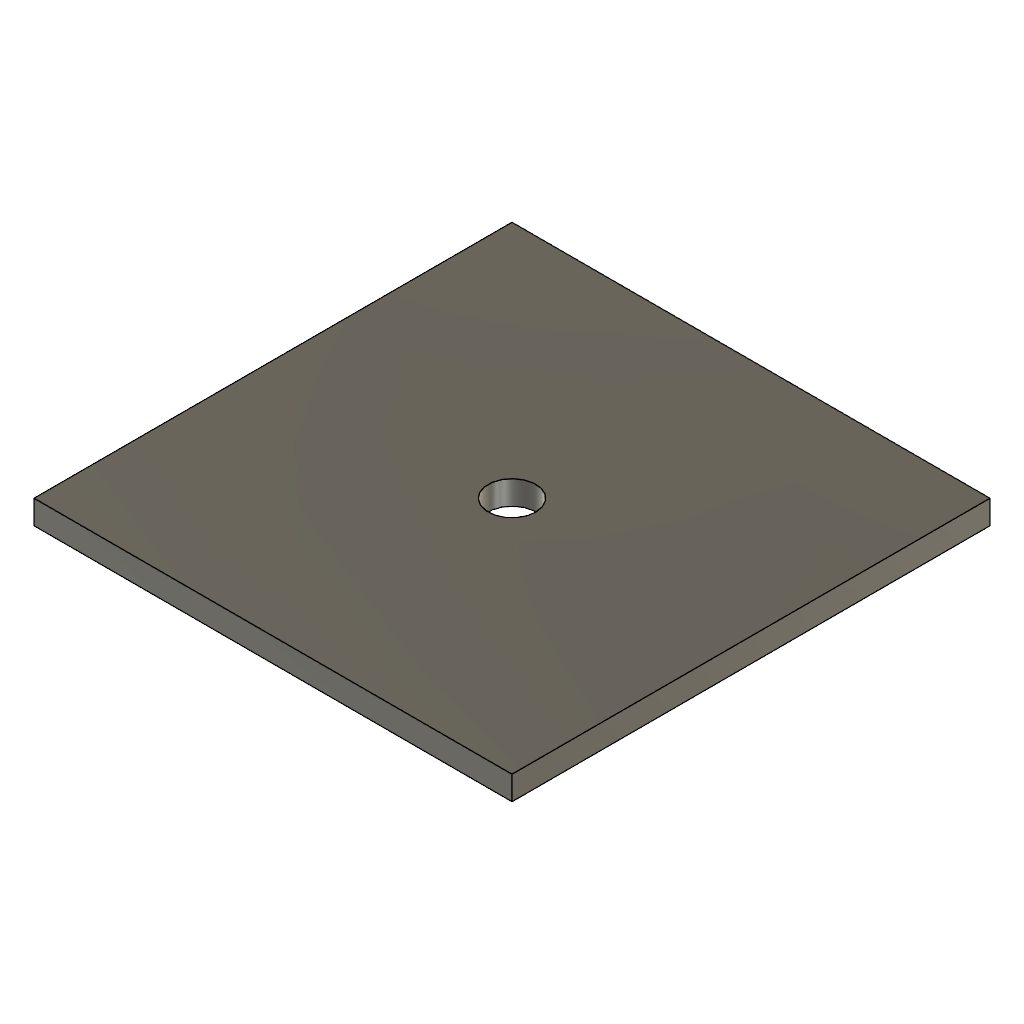
smart dice (Assembly) (Autodesk Fusion 360 archive; units mm, degrees)
design "steen ontwerp smart dice bovenkant"
Autodesk Fusion 360 part; units mm, degrees
sketch "Sketch1" plane through (0, 0, 0) normal (0, 0, 1) x (1, 0, 0)
  line L0 (-50, 50) -> (50, 50)
  line L1 (50, 50) -> (50, -50)
  line L2 (50, -50) -> (-50, -50)
  line L3 (-50, -50) -> (-50, 50)
  line L4 (-50, 50) -> (50, -50) construction
  line L5 (50, 50) -> (-50, -50) construction
  dimension "d1" = 100
  dimension "d2" = 100
  constraint horizontal L0
  constraint perpendicular L0 L1
  constraint parallel L0 L2
  constraint parallel L1 L3
  constraint coincident L4 origin
  constraint coincident L5 origin
  measures "d1" distance of L1.end L2.end
  measures "d2" distance of L0.end L1.end
extrude "Extrude1" add sketch "Sketch1" along normal blind 5
sketch "Sketch2" plane through (0, 0, 5) normal (0, 0, 1) x (-1, 0, 0)
  line L0 (50, 50) -> (-50, 50)
  line L1 (-50, 50) -> (-50, -50)
  line L2 (-50, -50) -> (50, -50)
  line L3 (50, -50) -> (50, 50)
  line L4 (40, -50) -> (40, 50) construction
  line L5 (30, -50) -> (30, 50) construction
  line L6 (20, 50) -> (20, -50) construction
  line L7 (10, -50) -> (10, 50) construction
  line L8 (0, 50) -> (0, -50) construction
  line L9 (-10, -50) -> (-10, 50) construction
  line L10 (-20, 50) -> (-20, -50) construction
  line L11 (-30, -50) -> (-30, 50) construction
  line L12 (-40, -50) -> (-40, 50) construction
  line L13 (-50, 40) -> (50, 40) construction
  line L14 (50, 30) -> (-50, 30) construction
  line L15 (-50, 20) -> (50, 20) construction
  line L16 (50, 10) -> (-50, 10) construction
  line L17 (-50, 0) -> (50, 0) construction
  line L18 (50, -10) -> (-50, -10) construction
  line L19 (-50, -20) -> (50, -20) construction
  line L20 (50, -30) -> (-50, -30) construction
  line L21 (-50, -40) -> (50, -40) construction
  circle A0 centre (0, 0) radius 5
  dimension "d5" = 10
  constraint coincident L2 L4.start
  constraint coincident L0 L4.end
  constraint perpendicular L0 L4
  constraint coincident L2 L5.start
  constraint coincident L0 L5.end
  constraint perpendicular L0 L5
  constraint coincident L0 L6.start
  constraint coincident L2 L6.end
  constraint perpendicular L2 L6
  constraint coincident L2 L7.start
  constraint coincident L0 L7.end
  constraint perpendicular L0 L7
  constraint midpoint L0 L8.start
  constraint midpoint L2 L8.end
  constraint coincident L2 L9.start
  constraint coincident L0 L9.end
  constraint perpendicular L0 L9
  constraint coincident L0 L10.start
  constraint coincident L2 L10.end
  constraint perpendicular L2 L10
  constraint coincident L2 L11.start
  constraint coincident L0 L11.end
  constraint perpendicular L0 L11
  constraint coincident L2 L12.start
  constraint coincident L0 L12.end
  constraint perpendicular L0 L12
  constraint coincident L1 L13.start
  constraint coincident L3 L13.end
  constraint perpendicular L3 L13
  constraint coincident L3 L14.start
  constraint coincident L1 L14.end
  constraint perpendicular L1 L14
  constraint coincident L1 L15.start
  constraint coincident L3 L15.end
  constraint perpendicular L3 L15
  constraint coincident L3 L16.start
  constraint coincident L1 L16.end
  constraint perpendicular L1 L16
  constraint midpoint L1 L17.start
  constraint midpoint L3 L17.end
  constraint coincident L3 L18.start
  constraint coincident L1 L18.end
  constraint perpendicular L1 L18
  constraint coincident L1 L19.start
  constraint coincident L3 L19.end
  constraint perpendicular L3 L19
  constraint coincident L3 L20.start
  constraint coincident L1 L20.end
  constraint perpendicular L1 L20
  constraint coincident L1 L21.start
  constraint coincident L3 L21.end
  constraint perpendicular L3 L21
  constraint coincident A0.centre origin
  measures "d5" diameter of A0
extrude "Extrude2" cut sketch "Sketch2" against normal blind 5 contours A0
sketch "Sketch3" plane through (0, 0, 0) normal (0, 0, -1) x (1, 0, 0)
  circle A0 centre (0, 0) radius 5
  line L0 (50, 50) -> (-50, 50)
  line L1 (-50, 50) -> (-50, -50)
  line L2 (-50, -50) -> (50, -50)
  line L3 (50, -50) -> (50, 50)
  line L4 (-50, 50) -> (-30, 50)
  line L5 (-30, -50) -> (-50, -50)
  line L6 (-50, -50) -> (-50, 50)
  line L7 (27.6819, -50) -> (50, -50)
  line L8 (50, -50) -> (50, 50)
  line L9 (50, 50) -> (27.6819, 50)
  line L10 (-40, 40) -> (-20, 40)
  line L11 (-20, 40) -> (-20, -40)
  line L12 (-20, -40) -> (-40, -40)
  line L13 (-40, -40) -> (-40, 40)
  line L14 (20, -40) -> (40, -40)
  line L15 (40, -40) -> (40, 40)
  line L16 (40, 40) -> (20, 40)
  line L17 (20, 40) -> (20, -40)
  constraint horizontal L4
  constraint horizontal L5
  constraint vertical L6
  constraint coincident L2 L5.start
  constraint coincident L0.end L1.start
  constraint horizontal L7
  constraint vertical L8
  constraint horizontal L9
  constraint coincident L0.start L3.end
  constraint coincident L2 L7.start
  constraint horizontal L10
  constraint vertical L11
  constraint horizontal L12
  constraint vertical L13
  constraint horizontal L14
  constraint vertical L15
  constraint horizontal L16
  constraint vertical L17
extrude "Extrude3" cut sketch "Sketch3" against normal blind 2 contours L10 L11 L12 L13 | L14 L15 L16 L17

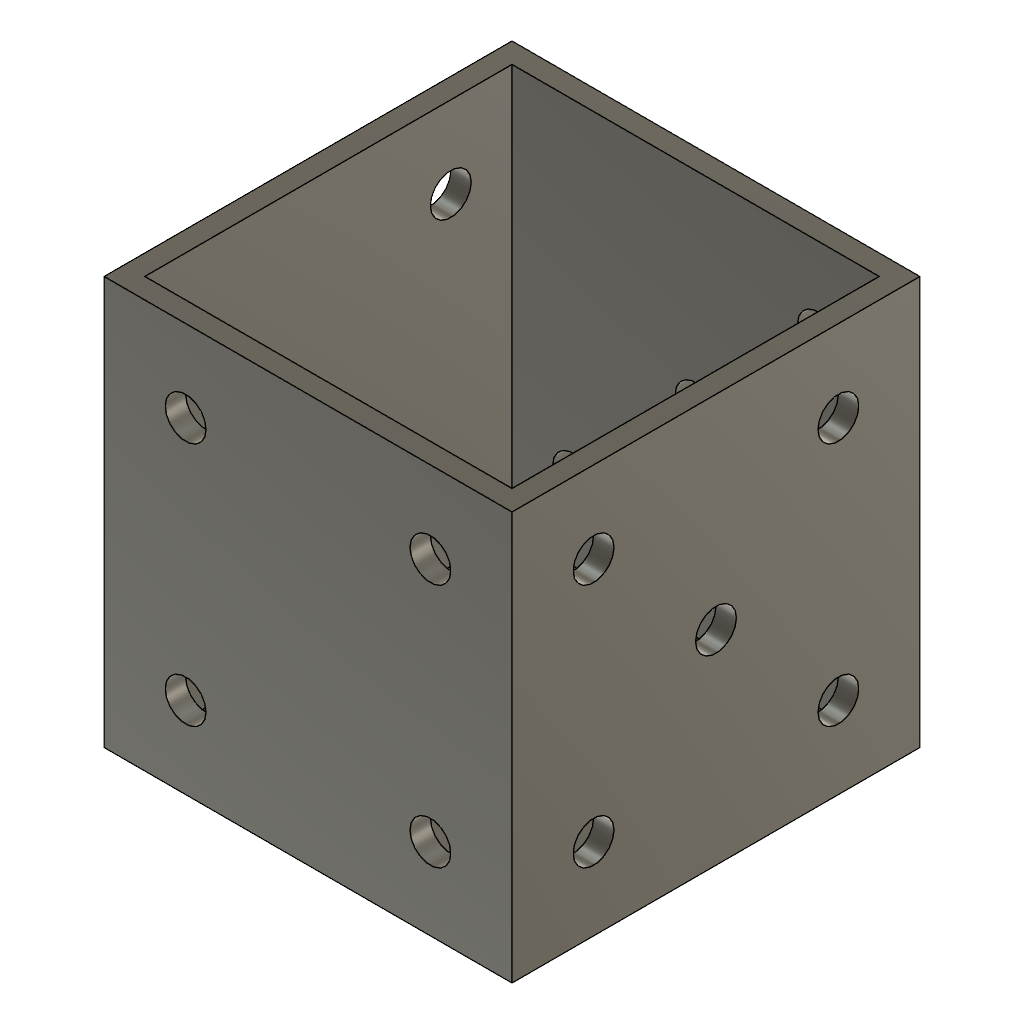
design "steen ontwerp smart dice onderkant"
Autodesk Fusion 360 part; units mm, degrees
sketch "Sketch1" plane through (0, 0, 0) normal (0, 0, 1) x (1, 0, 0)
  line L0 (-50, 50) -> (50, 50)
  line L1 (50, 50) -> (50, -50)
  line L2 (50, -50) -> (-50, -50)
  line L3 (-50, -50) -> (-50, 50)
  line L4 (-45, -45) -> (45, -45)
  line L5 (45, -45) -> (45, 45)
  line L6 (45, 45) -> (-45, 45)
  line L7 (-45, 45) -> (-45, -45)
  line L8 (-45, -45) -> (45, 45) construction
  line L9 (45, -45) -> (-45, 45) construction
  dimension "d5" = 90
  dimension "d6" = 90
  constraint horizontal L0
  constraint vertical L1
  constraint horizontal L2
  constraint vertical L3
  constraint horizontal L4
  constraint perpendicular L4 L5
  constraint parallel L4 L6
  constraint parallel L5 L7
  constraint coincident L8 origin
  constraint coincident L9 origin
  measures "d5" distance of L5.end L6.end
  measures "d6" distance of L4.end L5.end
extrude "Extrude3" add sketch "Sketch1" along normal blind 100
extrude "Extrude4" add sketch "Sketch1" along normal blind 1 contours L4 L5 L6 L7
sketch "Sketch3" plane through (50, 0, 0) normal (1, 0, 0) x (0, 1, 0)
  line L0 (-50, 0) -> (50, 0)
  line L1 (50, 0) -> (50, 100)
  line L2 (50, 100) -> (-50, 100)
  line L3 (-50, 100) -> (-50, 0)
  line L4 (-40, 100) -> (-40, 0) construction
  line L5 (-30, 100) -> (-30, 0) construction
  line L6 (-20, 100) -> (-20, 0) construction
  line L7 (-10, 100) -> (-10, 0) construction
  line L8 (10, 100) -> (10, 0) construction
  line L9 (20, 100) -> (20, 0) construction
  line L10 (30, 100) -> (30, 0) construction
  line L11 (40, 100) -> (40, 0) construction
  line L12 (-50, 10) -> (50, 10) construction
  line L13 (-50, 20) -> (50, 20) construction
  line L14 (-50, 30) -> (50, 30) construction
  line L15 (-50, 40) -> (50, 40) construction
  line L16 (-50, 50) -> (50, 50) construction
  line L17 (-50, 60) -> (50, 60) construction
  line L18 (-50, 70) -> (50, 70) construction
  line L19 (50, 80) -> (-50, 80) construction
  line L20 (-50, 90) -> (50, 90) construction
  line L21 (0, 100) -> (0, 0) construction
  circle A0 centre (-30, 80) radius 5
  circle A1 centre (30, 80) radius 5
  circle A2 centre (-30, 20) radius 5
  circle A3 centre (30, 20) radius 5
  circle A4 centre (0, 50) radius 5
  dimension "d12" = 10
  dimension "d13" = 10
  dimension "d14" = 10
  dimension "d15" = 10
  dimension "d16" = 10
  constraint coincident L2 L4.start
  constraint coincident L0 L4.end
  constraint perpendicular L0 L4
  constraint coincident L2 L5.start
  constraint coincident L0 L5.end
  constraint perpendicular L0 L5
  constraint coincident L2 L6.start
  constraint coincident L0 L6.end
  constraint perpendicular L0 L6
  constraint coincident L2 L7.start
  constraint coincident L0 L7.end
  constraint perpendicular L0 L7
  constraint coincident L2 L8.start
  constraint coincident L0 L8.end
  constraint perpendicular L0 L8
  constraint coincident L2 L9.start
  constraint coincident L0 L9.end
  constraint perpendicular L0 L9
  constraint coincident L2 L10.start
  constraint coincident L0 L10.end
  constraint perpendicular L0 L10
  constraint coincident L2 L11.start
  constraint coincident L0 L11.end
  constraint perpendicular L0 L11
  constraint coincident L3 L12.start
  constraint coincident L1 L12.end
  constraint perpendicular L1 L12
  constraint coincident L3 L13.start
  constraint coincident L1 L13.end
  constraint perpendicular L1 L13
  constraint coincident L3 L14.start
  constraint coincident L1 L14.end
  constraint perpendicular L1 L14
  constraint coincident L3 L15.start
  constraint coincident L1 L15.end
  constraint perpendicular L1 L15
  constraint midpoint L3 L16.start
  constraint midpoint L1 L16.end
  constraint coincident L3 L17.start
  constraint coincident L1 L17.end
  constraint perpendicular L1 L17
  constraint coincident L3 L18.start
  constraint coincident L1 L18.end
  constraint perpendicular L1 L18
  constraint coincident L1 L19.start
  constraint coincident L3 L19.end
  constraint perpendicular L3 L19
  constraint coincident L3 L20.start
  constraint coincident L1 L20.end
  constraint perpendicular L1 L20
  constraint midpoint L2 L21.start
  constraint coincident L21.end origin
  constraint coincident L19 A0.centre
  constraint coincident L5 A0.centre
  constraint coincident L10 A1.centre
  constraint coincident L19 A1.centre
  constraint coincident L5 A2.centre
  constraint coincident L13 A2.centre
  constraint coincident L10 A3.centre
  constraint coincident L13 A3.centre
  constraint midpoint L21 A4.centre
  measures "d12" diameter of A0
  measures "d13" diameter of A1
  measures "d14" diameter of A2
  measures "d15" diameter of A3
  measures "d16" diameter of A4
extrude "Extrude5" cut sketch "Sketch3" against normal blind 10 contours A0 | A1 | A2 | A3 | A4
sketch "Sketch4" plane through (-50, 0, 0) normal (-1, 0, 0) x (0, -1, 0)
  line L0 (-50, 0) -> (50, 0)
  line L1 (50, 0) -> (50, 100)
  line L2 (50, 100) -> (-50, 100)
  line L3 (-50, 100) -> (-50, 0)
  line L4 (-40, 100) -> (-40, 0) construction
  line L5 (-30, 0) -> (-30, 100) construction
  line L6 (-20, 100) -> (-20, 0) construction
  line L7 (-10, 0) -> (-10, 100) construction
  line L8 (0, 100) -> (0, 0) construction
  line L9 (10, 0) -> (10, 100) construction
  line L10 (20, 100) -> (20, 0) construction
  line L11 (30, 0) -> (30, 100) construction
  line L12 (40, 100) -> (40, 0) construction
  line L13 (50, 10) -> (-50, 10) construction
  line L14 (-50, 20) -> (50, 20) construction
  line L15 (50, 30) -> (-50, 30) construction
  line L16 (-50, 40) -> (50, 40) construction
  line L17 (50, 50) -> (-50, 50) construction
  line L18 (-50, 60) -> (50, 60) construction
  line L19 (50, 70) -> (-50, 70) construction
  line L20 (-50, 80) -> (50, 80) construction
  line L21 (50, 90) -> (-50, 90) construction
  circle A0 centre (-30, 80) radius 5
  circle A1 centre (30, 20) radius 5
  dimension "d19" = 10
  dimension "d20" = 10
  constraint coincident L2 L4.start
  constraint coincident L0 L4.end
  constraint perpendicular L0 L4
  constraint coincident L0 L5.start
  constraint coincident L2 L5.end
  constraint perpendicular L2 L5
  constraint coincident L2 L6.start
  constraint coincident L0 L6.end
  constraint perpendicular L0 L6
  constraint coincident L0 L7.start
  constraint coincident L2 L7.end
  constraint perpendicular L2 L7
  constraint midpoint L2 L8.start
  constraint coincident L8.end origin
  constraint coincident L0 L9.start
  constraint coincident L2 L9.end
  constraint perpendicular L2 L9
  constraint coincident L2 L10.start
  constraint coincident L0 L10.end
  constraint perpendicular L0 L10
  constraint coincident L0 L11.start
  constraint coincident L2 L11.end
  constraint perpendicular L2 L11
  constraint coincident L2 L12.start
  constraint coincident L0 L12.end
  constraint perpendicular L0 L12
  constraint coincident L1 L13.start
  constraint coincident L3 L13.end
  constraint perpendicular L3 L13
  constraint coincident L3 L14.start
  constraint coincident L1 L14.end
  constraint perpendicular L1 L14
  constraint coincident L1 L15.start
  constraint coincident L3 L15.end
  constraint perpendicular L3 L15
  constraint coincident L3 L16.start
  constraint coincident L1 L16.end
  constraint perpendicular L1 L16
  constraint midpoint L1 L17.start
  constraint midpoint L3 L17.end
  constraint coincident L3 L18.start
  constraint coincident L1 L18.end
  constraint perpendicular L1 L18
  constraint coincident L1 L19.start
  constraint coincident L3 L19.end
  constraint perpendicular L3 L19
  constraint coincident L3 L20.start
  constraint coincident L1 L20.end
  constraint perpendicular L1 L20
  constraint coincident L1 L21.start
  constraint coincident L3 L21.end
  constraint perpendicular L3 L21
  constraint coincident L20 A0.centre
  constraint coincident L5 A0.centre
  constraint coincident L11 A1.centre
  constraint coincident L14 A1.centre
  measures "d19" diameter of A0
  measures "d20" diameter of A1
extrude "Extrude6" cut sketch "Sketch4" against normal blind 10 contours A0
extrude "Extrude7" cut sketch "Sketch4" against normal blind 10 contours A1
sketch "Sketch5" plane through (0, 0, 0) normal (0, 0, -1) x (1, 0, 0)
  line L0 (50, 50) -> (-50, 50)
  line L1 (-50, 50) -> (-50, -50)
  line L2 (-50, -50) -> (50, -50)
  line L3 (50, -50) -> (50, 50)
  line L4 (-40, 50) -> (-40, -50) construction
  line L5 (-30, -50) -> (-30, 50) construction
  line L6 (-20, 50) -> (-20, -50) construction
  line L7 (-10, -50) -> (-10, 50) construction
  line L8 (0, 50) -> (0, -50) construction
  line L9 (10, -50) -> (10, 50) construction
  line L10 (20, 50) -> (20, -50) construction
  line L11 (30, -50) -> (30, 50) construction
  line L12 (40, 50) -> (40, -50) construction
  line L13 (50, -40) -> (-50, -40) construction
  line L14 (-50, -30) -> (50, -30) construction
  line L15 (50, -20) -> (-50, -20) construction
  line L16 (-50, -10) -> (50, -10) construction
  line L17 (50, 0) -> (-50, 0) construction
  line L18 (-50, 10) -> (50, 10) construction
  line L19 (50, 20) -> (-50, 20) construction
  line L20 (-50, 30) -> (50, 30) construction
  line L21 (-50, 40) -> (50, 40) construction
  circle A0 centre (-30, 30) radius 5
  circle A1 centre (30, 30) radius 5
  circle A2 centre (-30, 0) radius 5
  circle A3 centre (30, 0) radius 5
  circle A4 centre (-30, -30) radius 5
  circle A5 centre (30, -30) radius 5
  dimension "d25" = 10
  dimension "d26" = 10
  dimension "d27" = 10
  dimension "d28" = 10
  dimension "d29" = 10
  dimension "d30" = 10
  constraint coincident L0 L4.start
  constraint coincident L2 L4.end
  constraint perpendicular L2 L4
  constraint coincident L2 L5.start
  constraint coincident L0 L5.end
  constraint perpendicular L0 L5
  constraint coincident L0 L6.start
  constraint coincident L2 L6.end
  constraint perpendicular L2 L6
  constraint coincident L2 L7.start
  constraint coincident L0 L7.end
  constraint perpendicular L0 L7
  constraint midpoint L0 L8.start
  constraint midpoint L2 L8.end
  constraint coincident L2 L9.start
  constraint coincident L0 L9.end
  constraint perpendicular L0 L9
  constraint coincident L0 L10.start
  constraint coincident L2 L10.end
  constraint perpendicular L2 L10
  constraint coincident L2 L11.start
  constraint coincident L0 L11.end
  constraint perpendicular L0 L11
  constraint coincident L0 L12.start
  constraint coincident L2 L12.end
  constraint perpendicular L2 L12
  constraint coincident L3 L13.start
  constraint coincident L1 L13.end
  constraint perpendicular L1 L13
  constraint coincident L1 L14.start
  constraint coincident L3 L14.end
  constraint perpendicular L3 L14
  constraint coincident L3 L15.start
  constraint coincident L1 L15.end
  constraint perpendicular L1 L15
  constraint coincident L1 L16.start
  constraint coincident L3 L16.end
  constraint perpendicular L3 L16
  constraint midpoint L3 L17.start
  constraint midpoint L1 L17.end
  constraint coincident L1 L18.start
  constraint coincident L3 L18.end
  constraint perpendicular L3 L18
  constraint coincident L3 L19.start
  constraint coincident L1 L19.end
  constraint coincident L1 L20.start
  constraint coincident L3 L20.end
  constraint perpendicular L3 L20
  constraint coincident L1 L21.start
  constraint coincident L3 L21.end
  constraint perpendicular L3 L21
  constraint coincident L5 A0.centre
  constraint coincident L20 A0.centre
  constraint coincident L11 A1.centre
  constraint coincident L20 A1.centre
  constraint midpoint L5 A2.centre
  constraint midpoint L11 A3.centre
  constraint coincident L14 A4.centre
  constraint coincident L5 A4.centre
  constraint coincident L14 A5.centre
  constraint coincident L11 A5.centre
  measures "d25" diameter of A0
  measures "d26" diameter of A1
  measures "d27" diameter of A2
  measures "d28" diameter of A3
  measures "d29" diameter of A4
  measures "d30" diameter of A5
extrude "Extrude8" cut sketch "Sketch5" against normal blind 2 contours A0 | A1 | A2 | A3 | A4 | A5
sketch "Sketch7" plane through (0, -50, 0) normal (0, -1, 0) x (1, 0, 0)
  line L0 (-50, 0) -> (50, 0)
  line L1 (50, 0) -> (50, 100)
  line L2 (50, 100) -> (-50, 100)
  line L3 (-50, 100) -> (-50, 0)
  line L4 (-40, 100) -> (-40, 0) construction
  line L5 (-30, 0) -> (-30, 100) construction
  line L6 (-20, 100) -> (-20, 0) construction
  line L7 (-10, 0) -> (-10, 100) construction
  line L8 (0, 100) -> (0, 0) construction
  line L9 (10, 0) -> (10, 100) construction
  line L10 (20, 0) -> (20, 100) construction
  line L11 (30, 100) -> (30, 0) construction
  line L12 (40, 0) -> (40, 100) construction
  line L13 (-50, 10) -> (50, 10) construction
  line L14 (50, 20) -> (-50, 20) construction
  line L15 (-50, 30) -> (50, 30) construction
  line L16 (50, 40) -> (-50, 40) construction
  line L17 (-50, 50) -> (50, 50) construction
  line L18 (50, 60) -> (-50, 60) construction
  line L19 (-50, 70) -> (50, 70) construction
  line L20 (50, 80) -> (-50, 80) construction
  line L21 (-50, 90) -> (50, 90) construction
  circle A0 centre (-30, 80) radius 5
  circle A1 centre (-30, 20) radius 5
  circle A2 centre (30, 20) radius 5
  circle A3 centre (30, 80) radius 5
  dimension "d33" = 10
  dimension "d34" = 10
  dimension "d35" = 10
  dimension "d36" = 10
  constraint coincident L2 L4.start
  constraint coincident L0 L4.end
  constraint perpendicular L0 L4
  constraint coincident L0 L5.start
  constraint coincident L2 L5.end
  constraint perpendicular L2 L5
  constraint coincident L2 L6.start
  constraint coincident L0 L6.end
  constraint perpendicular L2 L6
  constraint coincident L0 L7.start
  constraint coincident L2 L7.end
  constraint perpendicular L2 L7
  constraint midpoint L2 L8.start
  constraint coincident L8.end origin
  constraint coincident L0 L9.start
  constraint coincident L2 L9.end
  constraint perpendicular L2 L9
  constraint coincident L0 L10.start
  constraint coincident L2 L10.end
  constraint coincident L2 L11.start
  constraint coincident L0 L11.end
  constraint perpendicular L0 L11
  constraint coincident L0 L12.start
  constraint coincident L2 L12.end
  constraint perpendicular L2 L12
  constraint coincident L3 L13.start
  constraint coincident L1 L13.end
  constraint perpendicular L1 L13
  constraint coincident L1 L14.start
  constraint coincident L3 L14.end
  constraint perpendicular L3 L14
  constraint coincident L3 L15.start
  constraint coincident L1 L15.end
  constraint perpendicular L1 L15
  constraint coincident L1 L16.start
  constraint coincident L3 L16.end
  constraint perpendicular L3 L16
  constraint midpoint L3 L17.start
  constraint midpoint L1 L17.end
  constraint coincident L1 L18.start
  constraint coincident L3 L18.end
  constraint perpendicular L3 L18
  constraint coincident L3 L19.start
  constraint coincident L1 L19.end
  constraint perpendicular L1 L19
  constraint coincident L1 L20.start
  constraint coincident L3 L20.end
  constraint perpendicular L3 L20
  constraint coincident L3 L21.start
  constraint coincident L1 L21.end
  constraint perpendicular L1 L21
  constraint coincident L20 A0.centre
  constraint coincident L5 A0.centre
  constraint coincident L14 A1.centre
  constraint coincident L5 A1.centre
  constraint coincident L14 A2.centre
  constraint coincident L11 A2.centre
  constraint coincident L11 A3.centre
  constraint coincident L20 A3.centre
  measures "d33" diameter of A0
  measures "d34" diameter of A1
  measures "d35" diameter of A2
  measures "d36" diameter of A3
extrude "Extrude9" cut sketch "Sketch7" against normal blind 5 contours A0 | A1 | A2 | A3
sketch "Sketch8" plane through (0, 50, 0) normal (0, 1, 0) x (-1, 0, 0)
  line L0 (-50, 0) -> (50, 0)
  line L1 (50, 0) -> (50, 100)
  line L2 (50, 100) -> (-50, 100)
  line L3 (-50, 100) -> (-50, 0)
  line L4 (-40, 100) -> (-40, 0) construction
  line L5 (-30, 0) -> (-30, 100) construction
  line L6 (-20, 100) -> (-20, 0) construction
  line L7 (-10, 0) -> (-10, 100) construction
  line L8 (0, 100) -> (0, 0) construction
  line L9 (10, 0) -> (10, 100) construction
  line L10 (20, 100) -> (20, 0) construction
  line L11 (30, 0) -> (30, 100) construction
  line L12 (40, 100) -> (40, 0) construction
  line L13 (-50, 10) -> (50, 10) construction
  line L14 (50, 20) -> (-50, 20) construction
  line L15 (-50, 30) -> (50, 30) construction
  line L16 (50, 40) -> (-50, 40) construction
  line L17 (-50, 50) -> (50, 50) construction
  line L18 (50, 60) -> (-50, 60) construction
  line L19 (-50, 70) -> (50, 70) construction
  line L20 (50, 80) -> (-50, 80) construction
  line L21 (-50, 90) -> (50, 90) construction
  circle A0 centre (-30, 80) radius 5
  circle A1 centre (0, 50) radius 5
  circle A2 centre (30, 20) radius 5
  dimension "d39" = 10
  dimension "d40" = 10
  dimension "d41" = 10
  constraint coincident L2 L4.start
  constraint coincident L0 L4.end
  constraint perpendicular L0 L4
  constraint coincident L0 L5.start
  constraint coincident L2 L5.end
  constraint perpendicular L2 L5
  constraint coincident L2 L6.start
  constraint coincident L0 L6.end
  constraint perpendicular L0 L6
  constraint coincident L0 L7.start
  constraint coincident L2 L7.end
  constraint perpendicular L2 L7
  constraint midpoint L2 L8.start
  constraint coincident L8.end origin
  constraint coincident L0 L9.start
  constraint coincident L2 L9.end
  constraint perpendicular L2 L9
  constraint coincident L2 L10.start
  constraint coincident L0 L10.end
  constraint perpendicular L0 L10
  constraint coincident L0 L11.start
  constraint coincident L2 L11.end
  constraint perpendicular L2 L11
  constraint coincident L2 L12.start
  constraint coincident L0 L12.end
  constraint perpendicular L0 L12
  constraint coincident L3 L13.start
  constraint coincident L1 L13.end
  constraint perpendicular L1 L13
  constraint coincident L1 L14.start
  constraint coincident L3 L14.end
  constraint perpendicular L3 L14
  constraint coincident L3 L15.start
  constraint coincident L1 L15.end
  constraint perpendicular L1 L15
  constraint coincident L1 L16.start
  constraint coincident L3 L16.end
  constraint perpendicular L3 L16
  constraint midpoint L3 L17.start
  constraint midpoint L1 L17.end
  constraint coincident L1 L18.start
  constraint coincident L3 L18.end
  constraint perpendicular L3 L18
  constraint coincident L3 L19.start
  constraint perpendicular L12 L19
  constraint coincident L1 L20.start
  constraint coincident L3 L20.end
  constraint perpendicular L3 L20
  constraint coincident L3 L21.start
  constraint coincident L1 L21.end
  constraint perpendicular L1 L21
  constraint coincident L5 A0.centre
  constraint coincident L20 A0.centre
  constraint midpoint L17 A1.centre
  constraint coincident L11 A2.centre
  constraint coincident L14 A2.centre
  measures "d39" diameter of A0
  measures "d40" diameter of A1
  measures "d41" diameter of A2
extrude "Extrude10" cut sketch "Sketch8" against normal blind 5 contours A0 | A1 | A2
